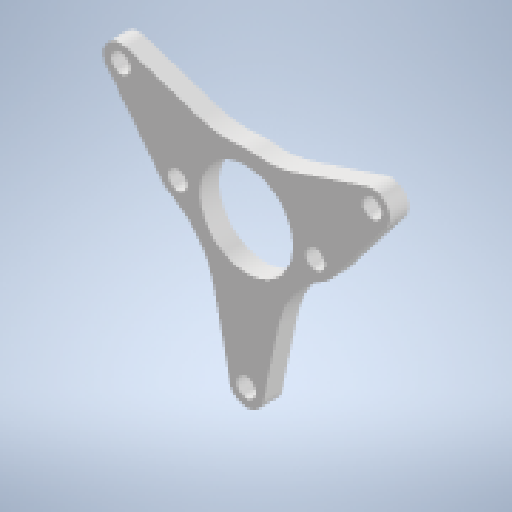
# Autodesk Inventor part: MotorHolder
Saved by Autodesk Inventor 2024 (Build 280153020, 153B)
## iProperties
Created: 2024-04-17
Part Number: MotorHolder
Material: Generic
Document SubType Name: Modeling
Designer: lvrectanus0
Density: 1 g/cm^3
Appearance: Default
Author: lvrectanus0
Autodesk Inventor part; units mm, degrees
ref_plane "YZ Plane" through (0, 0, 0) normal (1, 0, 0) x (0, 1, 0)
ref_plane "XZ Plane" through (0, 0, 0) normal (0, 1, 0) x (-1, 0, 0)
ref_plane "XY Plane" through (0, 0, 0) normal (0, 0, 1) x (1, 0, 0)
sketch "Sketch1" plane through (0, 0, 0) normal (0, 0, 1) x (1, 0, 0)
  circle A0 centre (8.9, 0) radius 18.65 projected
  circle A1 centre (23.4, 0) radius 1.65 projected
  circle A2 centre (-5.6, 0) radius 1.65 projected
  arc A3 (13.951, -13.4327) -> (21.5237, -6.826) centre (8.9, 0) ccw projected
  arc A4 (22.3604, -6.5571) -> (21.5237, -6.826) centre (22.0823, -7.128) ccw projected
  line L0 (22.3604, -6.5571) -> (23.5602, -7.1416) projected
  arc A5 (23.8417, -8.0126) -> (23.5602, -7.1416) centre (23.2821, -7.7125) ccw projected
  arc A6 (14.8123, -15.8902) -> (23.8417, -8.0126) centre (8.9, 0) ccw projected
  arc A7 (13.9876, -15.4932) -> (14.8123, -15.8902) centre (14.5909, -15.2951) ccw projected
  line L1 (13.9876, -15.4932) -> (13.5712, -14.2252) projected
  arc A8 (13.951, -13.4327) -> (13.5712, -14.2252) centre (14.1745, -14.0271) ccw projected
  line L2 (-4.5604, 6.5571) -> (-5.7602, 7.1416) projected
  arc A9 (-6.0417, 8.0126) -> (-5.7602, 7.1416) centre (-5.4821, 7.7125) ccw projected
  arc A10 (2.9877, 15.8902) -> (-6.0417, 8.0126) centre (8.9, 0) ccw projected
  arc A11 (3.8124, 15.4932) -> (2.9877, 15.8902) centre (3.2091, 15.2951) ccw projected
  line L3 (3.8124, 15.4932) -> (4.2288, 14.2252) projected
  arc A12 (3.849, 13.4327) -> (4.2288, 14.2252) centre (3.6255, 14.0271) ccw projected
  arc A13 (3.849, 13.4327) -> (-3.7237, 6.826) centre (8.9, 0) ccw projected
  arc A14 (-4.5604, 6.5571) -> (-3.7237, 6.826) centre (-4.2823, 7.128) ccw projected
  circle A15 centre (8.9, 0) radius 8.75 projected
  line L4 (22.3604, 6.5571) -> (23.5602, 7.1416) projected
  arc A16 (21.5237, 6.826) -> (22.3604, 6.5571) centre (22.0823, 7.128) ccw projected
  arc A17 (21.5237, 6.826) -> (13.951, 13.4327) centre (8.9, 0) ccw projected
  arc A18 (13.5712, 14.2252) -> (13.951, 13.4327) centre (14.1745, 14.0271) ccw projected
  line L5 (13.9876, 15.4932) -> (13.5712, 14.2252) projected
  arc A19 (14.8123, 15.8902) -> (13.9876, 15.4932) centre (14.5909, 15.2951) ccw projected
  arc A20 (23.8417, 8.0126) -> (14.8123, 15.8902) centre (8.9, 0) ccw projected
  arc A21 (23.5602, 7.1416) -> (23.8417, 8.0126) centre (23.2821, 7.7125) ccw projected
  line L6 (-4.5604, -6.5571) -> (-5.7602, -7.1416) projected
  arc A22 (-3.7237, -6.826) -> (-4.5604, -6.5571) centre (-4.2823, -7.128) ccw projected
  arc A23 (-3.7237, -6.826) -> (3.849, -13.4327) centre (8.9, 0) ccw projected
  arc A24 (4.2288, -14.2252) -> (3.849, -13.4327) centre (3.6255, -14.0271) ccw projected
  line L7 (3.8124, -15.4932) -> (4.2288, -14.2252) projected
  arc A25 (2.9877, -15.8902) -> (3.8124, -15.4932) centre (3.2091, -15.2951) ccw projected
  arc A26 (-6.0417, -8.0126) -> (2.9877, -15.8902) centre (8.9, 0) ccw projected
  arc A27 (-5.7602, -7.1416) -> (-6.0417, -8.0126) centre (-5.4821, -7.7125) ccw projected
  circle A28 centre (-5.6, 0) radius 1.65
  circle A29 centre (23.4, 0) radius 1.65
  circle A30 centre (8.9, 0) radius 9.75
  line L8 (8.9, 0) -> (8.9, -30.48)
  circle A31 centre (8.9, -30.48) radius 2
  circle A32 centre (8.9, -30.48) radius 3.6
  line L9 (5.374, -31.2064) -> (-0.6495, -1.9673)
  line L10 (12.426, -31.2064) -> (18.4495, -1.9673)
  circle A33 centre (35.2965, 15.24) radius 2
  circle A34 centre (35.2965, 15.24) radius 3.6
  line L11 (8.9, 0) -> (35.2965, 15.24)
  line L12 (34.1625, 18.6568) -> (5.829, 9.2537)
  line L13 (37.6885, 12.5496) -> (15.3784, -7.2864)
  circle A35 centre (-17.4965, 15.24) radius 2
  circle A36 centre (-17.4965, 15.24) radius 3.6
  line L14 (8.9, 0) -> (-17.4965, 15.24)
  line L15 (-19.8885, 12.5496) -> (2.4216, -7.2864)
  line L16 (-16.3625, 18.6568) -> (11.971, 9.2537)
  circle A37 centre (-5.6, 0) radius 2
  circle A38 centre (-5.6, 0) radius 3.6
  circle A39 centre (23.4, 0) radius 2
  circle A40 centre (23.4, 0) radius 3.6
  line L17 (0.0034, -5.1364) -> (-6.4857, -3.4893)
  line L18 (-19.8885, 12.5496) -> (-8.4448, -2.2062)
  line L19 (37.6885, 12.5496) -> (26.2448, -2.2062)
  line L20 (17.7966, -5.1364) -> (24.2857, -3.4893)
  circle A41 centre (8.9, 0) radius 12.85
  point P0 (0, 0)
  point P1 (15.6508, -15.5526)
  point P2 (16.3247, -12.2811)
  point P3 (8.9, 10.2729)
  point P4 (1.4753, -12.2811)
  point P5 (2.1492, -15.5526)
  point P6 (13.7731, 11.8901)
  point P7 (4.0269, 11.8901)
  point P8 (16.7606, -10.1653)
  point P9 (21.001, -4.3231)
  point P10 (-3.201, -4.3231)
  point P11 (1.0394, -10.1653)
  dimension "d0" = 1
  dimension "d1" = 4
  dimension "d2" = 7.2
  dimension "d3" = 30.48
  dimension "d6" = 360
  dimension "d8" = 4
  dimension "d9" = 7.2
  dimension "d10" = 4
  dimension "d11" = 7.2
  constraints: 26 end point, 14 centre point, 13 coincident, 12 point on circle, 9 tangent, 4 point on line, 2 concentric, 1 vertical, 40 other
  measures "d0" radial gap between concentric circles of A15 A30
  measures "d1" diameter of A31
  measures "d2" diameter of A32
  measures "d3" distance of L8.start L8.end
  measures "d8" diameter of A37
  measures "d9" diameter of A38
  measures "d10" diameter of A39
  measures "d11" diameter of A40
extrude "Extrusion1" add sketch "Sketch1" along normal blind 4 contours A0 L19 A40 L13 | A0 L13 L19 | L13 A40 A41 L11 A17 A16 L4 A21 A20 A0 | A0 L11 A34 L13 | L11 A20 L12 A0 | A0 L12 A34 L11 | A34 | A40 A41 L13 A39 | L13 A39 A41 A40 | L10 A32 L8 A0 | A0 L8 A41 L10 A3 A8 L1 A7 A6 | L11 A17 L12 A20 | A20 A21 L4 A16 A17 L11 | A41 A39 L13 A40 | A40 L13 L10 A30 L11 A41 | L8 A32 L9 A0 | A0 L9 A26 A25 L7 A24 A23 A41 L8 | A32 | A6 A7 L1 A8 A3 L10 | L20 A41 A40 | L16 A10 L14 A0 | A0 L14 A36 L16 | L11 A41 L12 A17 | A40 A41 L20 L13 | L13 A41 A40 | L11 A30 L16 L12 A41 | A41 L9 L15 A30 L8 | L8 A30 L13 L10 A41 | A41 L10 L20 | L14 A10 A9 L2 A14 A13 A41 A38 L15 A0 | A0 L15 A36 L14 | A36 | L16 A13 L14 A10 | L13 A41 A39 | L13 A30 L10 | L12 L16 A41 | L18 L15 A0 | A0 L15 A38 L18 | L9 A23 A24 L7 A25 A26 | A41 L17 L9 | L14 A13 A14 L2 A9 A10 | L16 A41 L14 A13 | A30 L12 L16 | L12 A30 L14 A41 L16 | A38 L15 A37 A41 | L15 L9 A30 | L15 A38 A41 L14 A30 L9 | L17 A41 A38 L15 | L17 A38 A41 | A38 A41 A37 L15 | A38 A41 L15 | L15 A41 A37 A38 | L15 A37 A41
fillet "Fillet1" radius 19.05 6 edges at (-3.201, -4.3231, 2) (1.0394, -10.1653, 2) (4.0269, 11.8901, 2) (13.7731, 11.8901, 2) (21.001, -4.3231, 2) (16.7606, -10.1653, 2)
sketch "Sketch2" plane through (0, 0, 4) normal (0, 0, 1) x (1, 0, 0)
  arc A0 (5.4731, -1.5453) -> (4.2552, -2.5573) centre (5.9714, -3.384) ccw projected
  arc A1 (4.2552, -2.5573) -> (4.6178, -3.1268) centre (8.9, 0) ccw projected
  arc A2 (4.6178, -3.1268) -> (6.05, -2.4513) centre (4.5948, -1.2219) ccw projected
  arc A3 (6.05, -2.4513) -> (6.7049, -3.0517) centre (8.9, 0) ccw projected
  arc A4 (6.7049, -3.0517) -> (6.1561, -4.5371) centre (8.0558, -4.3949) ccw projected
  arc A5 (6.1561, -4.5371) -> (6.7549, -4.849) centre (8.9, 0) ccw projected
  arc A6 (6.7549, -4.849) -> (7.6574, -3.5479) centre (5.7825, -3.2108) ccw projected
  arc A7 (7.6574, -3.5479) -> (8.5249, -3.7404) centre (8.9, 0) ccw projected
  arc A8 (8.5249, -3.7404) -> (8.7922, -5.3012) centre (10.3664, -4.2282) ccw projected
  arc A9 (8.7922, -5.3012) -> (9.4668, -5.2719) centre (8.9, 0) ccw projected
  arc A10 (9.4668, -5.2719) -> (9.5979, -3.6939) centre (7.8056, -4.3394) ccw projected
  arc A11 (9.5979, -3.6939) -> (10.4453, -3.4269) centre (8.9, 0) ccw projected
  arc A12 (10.4453, -3.4269) -> (11.4573, -4.6448) centre (12.284, -2.9286) ccw projected
  arc A13 (11.4573, -4.6448) -> (12.0268, -4.2822) centre (8.9, 0) ccw projected
  arc A14 (12.0268, -4.2822) -> (11.3513, -2.85) centre (10.1219, -4.3052) ccw projected
  arc A15 (11.3513, -2.85) -> (11.9517, -2.1951) centre (8.9, 0) ccw projected
  arc A16 (11.9517, -2.1951) -> (13.4371, -2.7439) centre (13.2949, -0.8442) ccw projected
  arc A17 (13.4371, -2.7439) -> (13.749, -2.1451) centre (8.9, 0) ccw projected
  arc A18 (13.749, -2.1451) -> (12.4479, -1.2426) centre (12.1108, -3.1175) ccw projected
  arc A19 (12.4479, -1.2426) -> (12.6404, -0.3751) centre (8.9, 0) ccw projected
  arc A20 (12.6404, -0.3751) -> (14.2012, -0.1078) centre (13.1282, 1.4664) ccw projected
  arc A21 (14.2012, -0.1078) -> (14.1719, 0.5668) centre (8.9, 0) ccw projected
  arc A22 (14.1719, 0.5668) -> (12.5939, 0.6979) centre (13.2394, -1.0944) ccw projected
  arc A23 (12.5939, 0.6979) -> (12.3269, 1.5453) centre (8.9, 0) ccw projected
  arc A24 (12.3269, 1.5453) -> (13.5448, 2.5573) centre (11.8286, 3.384) ccw projected
  arc A25 (13.5448, 2.5573) -> (13.1822, 3.1268) centre (8.9, 0) ccw projected
  arc A26 (13.1822, 3.1268) -> (11.75, 2.4513) centre (13.2052, 1.2219) ccw projected
  arc A27 (11.75, 2.4513) -> (11.0951, 3.0517) centre (8.9, 0) ccw projected
  arc A28 (11.0951, 3.0517) -> (11.6439, 4.5371) centre (9.7442, 4.3949) ccw projected
  arc A29 (11.6439, 4.5371) -> (11.0451, 4.849) centre (8.9, 0) ccw projected
  arc A30 (11.0451, 4.849) -> (10.1426, 3.5479) centre (12.0175, 3.2108) ccw projected
  arc A31 (10.1426, 3.5479) -> (9.2751, 3.7404) centre (8.9, 0) ccw projected
  arc A32 (9.2751, 3.7404) -> (9.0078, 5.3012) centre (7.4336, 4.2282) ccw projected
  arc A33 (9.0078, 5.3012) -> (8.3332, 5.2719) centre (8.9, 0) ccw projected
  arc A34 (8.3332, 5.2719) -> (8.2021, 3.6939) centre (9.9944, 4.3394) ccw projected
  arc A35 (8.2021, 3.6939) -> (7.3547, 3.4269) centre (8.9, 0) ccw projected
  arc A36 (7.3547, 3.4269) -> (6.3427, 4.6448) centre (5.516, 2.9286) ccw projected
  arc A37 (6.3427, 4.6448) -> (5.7732, 4.2822) centre (8.9, 0) ccw projected
  arc A38 (5.7732, 4.2822) -> (6.4487, 2.85) centre (7.6781, 4.3052) ccw projected
  arc A39 (6.4487, 2.85) -> (5.8483, 2.1951) centre (8.9, 0) ccw projected
  arc A40 (5.8483, 2.1951) -> (4.3629, 2.7439) centre (4.5051, 0.8442) ccw projected
  arc A41 (4.3629, 2.7439) -> (4.051, 2.1451) centre (8.9, 0) ccw projected
  arc A42 (4.051, 2.1451) -> (5.3521, 1.2426) centre (5.6892, 3.1175) ccw projected
  arc A43 (5.3521, 1.2426) -> (5.1596, 0.3751) centre (8.9, 0) ccw projected
  arc A44 (5.1596, 0.3751) -> (3.5988, 0.1078) centre (4.6718, -1.4664) ccw projected
  arc A45 (3.5988, 0.1078) -> (3.6281, -0.5668) centre (8.9, 0) ccw projected
  arc A46 (3.6281, -0.5668) -> (5.2061, -0.6979) centre (4.5606, 1.0944) ccw projected
  arc A47 (5.2061, -0.6979) -> (5.4731, -1.5453) centre (8.9, 0) ccw projected
  circle A48 centre (8.9, 0) radius 2.7343 projected
  circle A49 centre (8.9, 27.5717) radius 23.8125
  circle A50 centre (8.9, 0) radius 3.7592
  line L0 (4.1375, 24.8221) -> (4.1375, 30.3213)
  line L1 (4.1375, 30.3213) -> (8.9, 33.071)
  line L2 (8.9, 33.071) -> (13.6625, 30.3213)
  line L3 (13.6625, 30.3213) -> (13.6625, 24.8221)
  line L4 (13.6625, 24.8221) -> (8.9, 22.0724)
  line L5 (8.9, 22.0724) -> (4.1375, 24.8221)
  line L6 (13.6625, 24.8221) -> (4.1375, 30.3213)
  line L7 (8.9, 33.071) -> (8.9, 22.0724)
  line L8 (4.1375, 24.8221) -> (13.6625, 30.3213)
  point P0 (0, 0)
  dimension "d15" = 47.625
  dimension "d16" = 9.525
  dimension "d17" = 9.525
  dimension "d18" = 9.525
  constraints: 18 end point, 3 equal length, 2 centre point, 2 coincident, 2 tangent, 1 midpoint, 1 parallel, 1 vertical, 1 vertical alignment
  measures "d15" diameter of A49
  measures "d16" distance between parallel lines of L3 L0
  measures "d17" distance between parallel lines of L2 L5
  measures "d18" distance between parallel lines of L4 L1
body "Solid1"
